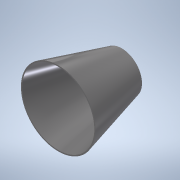
# Autodesk Inventor part: Redukcja symetryczna Ø129x70x2 L=110
Saved by Autodesk Inventor 2020 (Build 240168000, 168)
## iProperties
RuleStatus: InUse
Created: 2022-03-21
Part Number: Redukcja symetryczna Ø129x70x2 L=110
Material: 304
Description: Redukcja symetryczna Ø129x70x2 L=110
Document SubType Name: Modelowanie
Designer: Radosław
Density: 8 g/cm^3
Sheet Metal Rule: 1,5
Sheet Metal Width: 0,000 mm
Sheet Metal Length: 0,000 mm
Sheet Metal Area: 0,000 mm^2
Appearance: Częściowo polerowany(1)
Author: Radosław
Autodesk Inventor part; units mm, degrees
ref_plane "YZ Plane" through (0, 0, 0) normal (1, 0, 0) x (0, 1, 0)
ref_plane "XY Plane" through (0, 0, 0) normal (0, 0, 1) x (1, 0, 0)
sketch "Szkic6" plane through (0, 0, 0) normal (0, 1, 0) x (-1, 0, 0)
  circle A0 centre (0, 0) radius 64.5
  dimension "d33" = 129
  constraints: 1 centre point, 1 coincident
  measures "d33" diameter of A0
ref_plane "Płaszczyzna konstrukcyjna1" through (0, 110, 0) normal (0, 1, 0) x (-1, 0, 0)
sketch "Szkic7" plane through (0, 110, 0) normal (0, 1, 0) x (-1, 0, 0)
  circle A0 centre (0, 0) radius 35
  dimension "d35" = 70
  constraints: 1 centre point, 1 coincident
  measures "d35" diameter of A0
loft "Wyciągnięcie złożone1" add profiles "Szkic6", "Szkic7"
shell "Skorupa1" thickness 2 removed faces 2 at (1.9985, 110, 11.019) at (-10.0865, 0, -16.1433)
equation "\"d33\" = OD1"
equation "\"d35\" = OD2"
equation "\"d52\" = THK"
equation "\"SzerokośćGięciaPodcięcia\" = Grubość"
equation "\"RozmiarPodcięciaNarożnika\" = 4 * Grubość"
equation "\"PromieńPrzejścia\" = PromieńGięcia"
equation "\"Rozmiar_promienia_Jacobiego\" = PromieńGięcia"
equation "\"Wielk_odstępu\" = Grubość"
equation "\"d2\" = PromieńGięcia"
equation "\"d23\" = PromieńGięcia"
equation "\"OD1\" = 129"
equation "\"OD2\" = 70"
equation "\"THK\" = 2"
equation "\"Grubość\" = 1.5"
equation "\"PromieńGięcia\" = 3"
